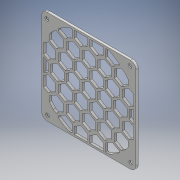
# Autodesk Inventor part: 120mm-honeycomb
Saved by Autodesk Inventor 2018 (Build 220112000, 112)
## iProperties
Created: 2017-10-04
Part Number: 120mm-honeycomb
Material: Generic
Document SubType Name: Modeling
Designer: leo2a
Density: 1 g/cm^3
Appearance: Default
Author: leo2a
Autodesk Inventor part; units mm, degrees
ref_plane "YZ Plane" through (0, 0, 0) normal (1, 0, 0) x (0, 1, 0)
ref_plane "XZ Plane" through (0, 0, 0) normal (0, 1, 0) x (-1, 0, 0)
ref_plane "XY Plane" through (0, 0, 0) normal (0, 0, 1) x (1, 0, 0)
sketch "Sketch1" plane through (0, 0, 0) normal (0, 1, 0) x (-1, 0, 0)
  line L0 (-60, 60) -> (-60, -60)
  line L1 (-60, -60) -> (60, -60)
  line L2 (60, -60) -> (60, 60)
  line L3 (60, 60) -> (-60, 60)
  arc A0 (24.4949, -57.5) -> (57.5, -24.4949) centre (0, 0) ccw
  line L4 (24.4949, -57.5) -> (-24.4949, -57.5)
  arc A1 (57.5, 24.4949) -> (24.4949, 57.5) centre (0, 0) ccw
  line L5 (57.5, 24.4949) -> (57.5, -24.4949)
  line L6 (-24.4949, 57.5) -> (24.4949, 57.5)
  arc A2 (-24.4949, 57.5) -> (-57.5, 24.4949) centre (0, 0) ccw
  arc A3 (-57.5, -24.4949) -> (-24.4949, -57.5) centre (0, 0) ccw
  line L7 (-57.5, -24.4949) -> (-57.5, 24.4949)
  point P0 (52.5, -52.5)
  point P1 (52.5, 52.5)
  point P2 (-52.5, 52.5)
  point P3 (-52.5, -52.5)
  dimension "d7" = 360
  constraints: 16 end point, 8 point on circle, 4 centre point, 4 parallel, 2 perpendicular, 1 coincident, 1 vertical, 5 other
extrude "Extrusion1" add sketch "Sketch1" along normal blind 3
sketch "Sketch2" plane through (0, 3, 0) normal (0, 1, 0) x (1, 0, 0)
  point P0 (0, 0)
  point P1 (-52.5, 53.5)
  point P2 (-53.5, -52.5)
  point P3 (52.5, -53.5)
  point P4 (53.5, 52.5)
  dimension "d17" = 360
  constraints: 5 other
hole "Hole1" at (-52.5, 3, -53.5) at (-53.5, 3, 52.5) at (52.5, 3, 53.5) at (53.5, 3, -52.5) direction (0, -1, 0) diameter 4.8 end through all counterbore diameter 8 counterbore depth 1.5 clearance for "Socket Head Cap Screw" size "M4" standard "Ansi Metric M Profile"
sketch "Sketch4" plane through (0, 0, 0) normal (0, 1, 0) x (-1, 0, 0)
  line L0 (0, -10) -> (-8.6603, -5)
  line L1 (-8.6603, -5) -> (-8.6603, 5)
  line L2 (-8.6603, 5) -> (0, 10)
  line L3 (0, 10) -> (8.6603, 5)
  line L4 (8.6603, 5) -> (8.6603, -5)
  line L5 (8.6603, -5) -> (0, -10)
  line L6 (0, 0) -> (-8.6603, 0)
  line L7 (0, 0) -> (-4.3301, -7.5)
  line L8 (10, -27.3205) -> (1.3397, -22.3205)
  line L9 (1.3397, -22.3205) -> (1.3397, -12.3205)
  line L10 (1.3397, -12.3205) -> (10, -7.3205)
  line L11 (10, -7.3205) -> (18.6603, -12.3205)
  line L12 (18.6603, -12.3205) -> (18.6603, -22.3205)
  line L13 (18.6603, -22.3205) -> (10, -27.3205)
  line L14 (11.3397, 5) -> (20, 10)
  line L15 (11.3397, -5) -> (11.3397, 5)
  line L16 (20, -10) -> (11.3397, -5)
  line L17 (28.6603, -5) -> (20, -10)
  line L18 (28.6603, 5) -> (28.6603, -5)
  line L19 (20, 10) -> (28.6603, 5)
  line L20 (1.3397, 12.3205) -> (1.3397, 22.3205)
  line L21 (10, 7.3205) -> (1.3397, 12.3205)
  line L22 (18.6603, 12.3205) -> (10, 7.3205)
  line L23 (18.6603, 22.3205) -> (18.6603, 12.3205)
  line L24 (10, 27.3205) -> (18.6603, 22.3205)
  line L25 (1.3397, 22.3205) -> (10, 27.3205)
  line L26 (-10, 7.3205) -> (-18.6603, 12.3205)
  line L27 (-1.3397, 12.3205) -> (-10, 7.3205)
  line L28 (-1.3397, 22.3205) -> (-1.3397, 12.3205)
  line L29 (-10, 27.3205) -> (-1.3397, 22.3205)
  line L30 (-18.6603, 22.3205) -> (-10, 27.3205)
  line L31 (-18.6603, 12.3205) -> (-18.6603, 22.3205)
  line L32 (-11.3397, -5) -> (-20, -10)
  line L33 (-11.3397, 5) -> (-11.3397, -5)
  line L34 (-20, 10) -> (-11.3397, 5)
  line L35 (-28.6603, 5) -> (-20, 10)
  line L36 (-28.6603, -5) -> (-28.6603, 5)
  line L37 (-20, -10) -> (-28.6603, -5)
  line L38 (-1.3397, -12.3205) -> (-1.3397, -22.3205)
  line L39 (-10, -7.3205) -> (-1.3397, -12.3205)
  line L40 (-18.6603, -12.3205) -> (-10, -7.3205)
  line L41 (-18.6603, -22.3205) -> (-18.6603, -12.3205)
  line L42 (-10, -27.3205) -> (-18.6603, -22.3205)
  line L43 (-1.3397, -22.3205) -> (-10, -27.3205)
  line L44 (38.6603, -12.3205) -> (38.6603, -22.3205)
  line L45 (38.6603, -22.3205) -> (30, -27.3205)
  line L46 (30, -27.3205) -> (21.3397, -22.3205)
  line L47 (21.3397, -22.3205) -> (21.3397, -12.3205)
  line L48 (21.3397, -12.3205) -> (30, -7.3205)
  line L49 (30, -7.3205) -> (38.6603, -12.3205)
  line L50 (21.3397, 22.3205) -> (30, 27.3205)
  line L51 (21.3397, 12.3205) -> (21.3397, 22.3205)
  line L52 (30, 7.3205) -> (21.3397, 12.3205)
  line L53 (38.6603, 12.3205) -> (30, 7.3205)
  line L54 (38.6603, 22.3205) -> (38.6603, 12.3205)
  line L55 (30, 27.3205) -> (38.6603, 22.3205)
  line L56 (-8.6603, 29.641) -> (-8.6603, 39.641)
  line L57 (0, 24.641) -> (-8.6603, 29.641)
  line L58 (8.6603, 29.641) -> (0, 24.641)
  line L59 (8.6603, 39.641) -> (8.6603, 29.641)
  line L60 (0, 44.641) -> (8.6603, 39.641)
  line L61 (-8.6603, 39.641) -> (0, 44.641)
  line L62 (-30, 7.3205) -> (-38.6603, 12.3205)
  line L63 (-21.3397, 12.3205) -> (-30, 7.3205)
  line L64 (-21.3397, 22.3205) -> (-21.3397, 12.3205)
  line L65 (-30, 27.3205) -> (-21.3397, 22.3205)
  line L66 (-38.6603, 22.3205) -> (-30, 27.3205)
  line L67 (-38.6603, 12.3205) -> (-38.6603, 22.3205)
  line L68 (-21.3397, -22.3205) -> (-30, -27.3205)
  line L69 (-21.3397, -12.3205) -> (-21.3397, -22.3205)
  line L70 (-30, -7.3205) -> (-21.3397, -12.3205)
  line L71 (-38.6603, -12.3205) -> (-30, -7.3205)
  line L72 (-38.6603, -22.3205) -> (-38.6603, -12.3205)
  line L73 (-30, -27.3205) -> (-38.6603, -22.3205)
  line L74 (8.6603, -29.641) -> (8.6603, -39.641)
  line L75 (0, -24.641) -> (8.6603, -29.641)
  line L76 (-8.6603, -29.641) -> (0, -24.641)
  line L77 (-8.6603, -39.641) -> (-8.6603, -29.641)
  line L78 (0, -44.641) -> (-8.6603, -39.641)
  line L79 (8.6603, -39.641) -> (0, -44.641)
  line L80 (28.6603, -29.641) -> (28.6603, -39.641)
  line L81 (28.6603, -39.641) -> (20, -44.641)
  line L82 (20, -44.641) -> (11.3397, -39.641)
  line L83 (11.3397, -39.641) -> (11.3397, -29.641)
  line L84 (11.3397, -29.641) -> (20, -24.641)
  line L85 (20, -24.641) -> (28.6603, -29.641)
  line L86 (31.3397, 5) -> (40, 10)
  line L87 (31.3397, -5) -> (31.3397, 5)
  line L88 (40, -10) -> (31.3397, -5)
  line L89 (48.6603, -5) -> (40, -10)
  line L90 (48.6603, 5) -> (48.6603, -5)
  line L91 (40, 10) -> (48.6603, 5)
  line L92 (11.3397, 29.641) -> (11.3397, 39.641)
  line L93 (20, 24.641) -> (11.3397, 29.641)
  line L94 (28.6603, 29.641) -> (20, 24.641)
  line L95 (28.6603, 39.641) -> (28.6603, 29.641)
  line L96 (20, 44.641) -> (28.6603, 39.641)
  line L97 (11.3397, 39.641) -> (20, 44.641)
  line L98 (-20, 24.641) -> (-28.6603, 29.641)
  line L99 (-11.3397, 29.641) -> (-20, 24.641)
  line L100 (-11.3397, 39.641) -> (-11.3397, 29.641)
  line L101 (-20, 44.641) -> (-11.3397, 39.641)
  line L102 (-28.6603, 39.641) -> (-20, 44.641)
  line L103 (-28.6603, 29.641) -> (-28.6603, 39.641)
  line L104 (-31.3397, -5) -> (-40, -10)
  line L105 (-31.3397, 5) -> (-31.3397, -5)
  line L106 (-40, 10) -> (-31.3397, 5)
  line L107 (-48.6603, 5) -> (-40, 10)
  line L108 (-48.6603, -5) -> (-48.6603, 5)
  line L109 (-40, -10) -> (-48.6603, -5)
  line L110 (-11.3397, -29.641) -> (-11.3397, -39.641)
  line L111 (-20, -24.641) -> (-11.3397, -29.641)
  line L112 (-28.6603, -29.641) -> (-20, -24.641)
  line L113 (-28.6603, -39.641) -> (-28.6603, -29.641)
  line L114 (-20, -44.641) -> (-28.6603, -39.641)
  line L115 (-11.3397, -39.641) -> (-20, -44.641)
  line L116 (18.6603, -48.5085) -> (18.6603, -58.5085)
  line L117 (10, -43.5085) -> (18.6603, -48.5085)
  line L118 (1.3397, -48.5085) -> (10, -43.5085)
  line L119 (1.3397, -58.5085) -> (1.3397, -48.5085)
  line L120 (10, -63.5085) -> (1.3397, -58.5085)
  line L121 (18.6603, -58.5085) -> (10, -63.5085)
  line L122 (-1.3397, -48.5085) -> (-1.3397, -58.5085)
  line L123 (-10, -43.5085) -> (-1.3397, -48.5085)
  line L124 (-18.6603, -48.5085) -> (-10, -43.5085)
  line L125 (-18.6603, -58.5085) -> (-18.6603, -48.5085)
  line L126 (-10, -63.5085) -> (-18.6603, -58.5085)
  line L127 (-1.3397, -58.5085) -> (-10, -63.5085)
  line L128 (32.6795, -30.4145) -> (41.3397, -25.4145)
  line L129 (32.6795, -40.4145) -> (32.6795, -30.4145)
  line L130 (41.3397, -45.4145) -> (32.6795, -40.4145)
  line L131 (50, -40.4145) -> (41.3397, -45.4145)
  line L132 (50, -30.4145) -> (50, -40.4145)
  line L133 (41.3397, -25.4145) -> (50, -30.4145)
  line L134 (42.6795, 13.094) -> (42.6795, 23.094)
  line L135 (51.3397, 8.094) -> (42.6795, 13.094)
  line L136 (60, 13.094) -> (51.3397, 8.094)
  line L137 (60, 23.094) -> (60, 13.094)
  line L138 (51.3397, 28.094) -> (60, 23.094)
  line L139 (42.6795, 23.094) -> (51.3397, 28.094)
  line L140 (10, 43.5085) -> (1.3397, 48.5085)
  line L141 (18.6603, 48.5085) -> (10, 43.5085)
  line L142 (18.6603, 58.5085) -> (18.6603, 48.5085)
  line L143 (10, 63.5085) -> (18.6603, 58.5085)
  line L144 (1.3397, 58.5085) -> (10, 63.5085)
  line L145 (1.3397, 48.5085) -> (1.3397, 58.5085)
  line L146 (-32.6795, 30.4145) -> (-41.3397, 25.4145)
  line L147 (-32.6795, 40.4145) -> (-32.6795, 30.4145)
  line L148 (-41.3397, 45.4145) -> (-32.6795, 40.4145)
  line L149 (-50, 40.4145) -> (-41.3397, 45.4145)
  line L150 (-50, 30.4145) -> (-50, 40.4145)
  line L151 (-41.3397, 25.4145) -> (-50, 30.4145)
  line L152 (-42.6795, -13.094) -> (-42.6795, -23.094)
  line L153 (-51.3397, -8.094) -> (-42.6795, -13.094)
  line L154 (-60, -13.094) -> (-51.3397, -8.094)
  line L155 (-60, -23.094) -> (-60, -13.094)
  line L156 (-51.3397, -28.094) -> (-60, -23.094)
  line L157 (-42.6795, -23.094) -> (-51.3397, -28.094)
  line L158 (42.6795, -13.094) -> (51.3397, -8.094)
  line L159 (51.3397, -28.094) -> (42.6795, -23.094)
  line L160 (42.6795, -23.094) -> (42.6795, -13.094)
  line L161 (60, -23.094) -> (51.3397, -28.094)
  line L162 (60, -13.094) -> (60, -23.094)
  line L163 (51.3397, -8.094) -> (60, -13.094)
  line L164 (32.6795, 30.4145) -> (32.6795, 40.4145)
  line L165 (50, 30.4145) -> (41.3397, 25.4145)
  line L166 (41.3397, 25.4145) -> (32.6795, 30.4145)
  line L167 (50, 40.4145) -> (50, 30.4145)
  line L168 (41.3397, 45.4145) -> (50, 40.4145)
  line L169 (32.6795, 40.4145) -> (41.3397, 45.4145)
  line L170 (-10, 43.5085) -> (-18.6603, 48.5085)
  line L171 (-1.3397, 58.5085) -> (-1.3397, 48.5085)
  line L172 (-1.3397, 48.5085) -> (-10, 43.5085)
  line L173 (-10, 63.5085) -> (-1.3397, 58.5085)
  line L174 (-18.6603, 58.5085) -> (-10, 63.5085)
  line L175 (-18.6603, 48.5085) -> (-18.6603, 58.5085)
  line L176 (-42.6795, 13.094) -> (-51.3397, 8.094)
  line L177 (-51.3397, 28.094) -> (-42.6795, 23.094)
  line L178 (-42.6795, 23.094) -> (-42.6795, 13.094)
  line L179 (-60, 23.094) -> (-51.3397, 28.094)
  line L180 (-60, 13.094) -> (-60, 23.094)
  line L181 (-51.3397, 8.094) -> (-60, 13.094)
  line L182 (-32.6795, -30.4145) -> (-32.6795, -40.4145)
  line L183 (-50, -30.4145) -> (-41.3397, -25.4145)
  line L184 (-41.3397, -25.4145) -> (-32.6795, -30.4145)
  line L185 (-50, -40.4145) -> (-50, -30.4145)
  line L186 (-41.3397, -45.4145) -> (-50, -40.4145)
  line L187 (-32.6795, -40.4145) -> (-41.3397, -45.4145)
  line L188 (30, -41.9615) -> (38.6603, -46.9615)
  line L189 (21.3397, -46.9615) -> (30, -41.9615)
  line L190 (21.3397, -56.9615) -> (21.3397, -46.9615)
  line L191 (30, -61.9615) -> (21.3397, -56.9615)
  line L192 (38.6603, -56.9615) -> (30, -61.9615)
  line L193 (38.6603, -46.9615) -> (38.6603, -56.9615)
  line L194 (51.3397, 5) -> (60, 10)
  line L195 (51.3397, -5) -> (51.3397, 5)
  line L196 (60, -10) -> (51.3397, -5)
  line L197 (68.6603, -5) -> (60, -10)
  line L198 (68.6603, 5) -> (68.6603, -5)
  line L199 (60, 10) -> (68.6603, 5)
  line L200 (21.3397, 46.9615) -> (21.3397, 56.9615)
  line L201 (30, 41.9615) -> (21.3397, 46.9615)
  line L202 (38.6603, 46.9615) -> (30, 41.9615)
  line L203 (38.6603, 56.9615) -> (38.6603, 46.9615)
  line L204 (30, 61.9615) -> (38.6603, 56.9615)
  line L205 (21.3397, 56.9615) -> (30, 61.9615)
  line L206 (-30, 41.9615) -> (-38.6603, 46.9615)
  line L207 (-21.3397, 46.9615) -> (-30, 41.9615)
  line L208 (-21.3397, 56.9615) -> (-21.3397, 46.9615)
  line L209 (-30, 61.9615) -> (-21.3397, 56.9615)
  line L210 (-38.6603, 56.9615) -> (-30, 61.9615)
  line L211 (-38.6603, 46.9615) -> (-38.6603, 56.9615)
  line L212 (-51.3397, -5) -> (-60, -10)
  line L213 (-51.3397, 5) -> (-51.3397, -5)
  line L214 (-60, 10) -> (-51.3397, 5)
  line L215 (-68.6603, 5) -> (-60, 10)
  line L216 (-68.6603, -5) -> (-68.6603, 5)
  line L217 (-60, -10) -> (-68.6603, -5)
  line L218 (-21.3397, -46.9615) -> (-21.3397, -56.9615)
  line L219 (-30, -41.9615) -> (-21.3397, -46.9615)
  line L220 (-38.6603, -46.9615) -> (-30, -41.9615)
  line L221 (-38.6603, -56.9615) -> (-38.6603, -46.9615)
  line L222 (-30, -61.9615) -> (-38.6603, -56.9615)
  line L223 (-21.3397, -56.9615) -> (-30, -61.9615)
  circle A0 centre (0, 0) radius 68.8421
  dimension "d39" = 10
  dimension "d42" = 360
  dimension "d48" = 360
  dimension "d56" = 360
  dimension "d72" = 360
  dimension "d76" = 360
  dimension "d90" = 360
  constraints: 448 end point, 2 midpoint, 1 coincident, 454 other
  measures "d39" distance of point (0, 0) L0.start
extrude "Extrusion2" add sketch "Sketch4" along normal blind 3 contours L189 L190 L191 A0 L223 L218 L219 L220 L221 L217 L212 L213 L214 L215 L211 L206 L207 L208 L209 L205 L200 L201 L202 L203 L199 L194 L195 L196 L197 L193 L188 | A0 L192 | L198 A0 | A0 L222 | L204 A0 | A0 L216 | L210 A0
sketch "Sketch5" plane through (0, 0, 0) normal (0, -1, 0) x (1, 0, 0)
  line L0 (-33.7525, -60) -> (-60, -60) projected
  line L1 (60, 60) -> (-60, 60)
  line L2 (-60, 60) -> (-60, -60)
  line L3 (-60, -60) -> (60, -60)
  line L4 (60, -60) -> (60, 60)
  line L5 (60, 60) -> (-60, -60) construction
  line L6 (-60, 60) -> (60, -60) construction
  line L7 (-70, 70) -> (70, 70)
  line L8 (70, 70) -> (70, -70)
  line L9 (70, -70) -> (-70, -70)
  line L10 (-70, -70) -> (-70, 70)
  point P0 (0, 0)
  dimension "d94" = 10
  constraints: 20 end point, 4 parallel, 2 midpoint, 2 perpendicular, 1 horizontal, 3 other
  measures "d94" distance between parallel lines of L1 L7
extrude "Extrusion3" cut sketch "Sketch5" against normal blind 5
fillet "Fillet1" radius 7 4 edges at (60, 1.5, 60) (60, 1.5, -60) (-60, 1.5, 60) (-60, 1.5, -60)
body "Solid1"
